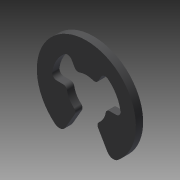
# Autodesk Inventor part: D-5406
Saved by Autodesk Inventor 2014 (Build 180170000, 170)
## iProperties
Created: 2014-01-19
Part Number: D-5406
Material: Generic
Catalog Web Link: www.cadenas.de
Description: Piston Rod Clevis for Original Line Cylinders - Retaining Ring-
Vendor: BIMBA
Document SubType Name: Standard Catalog Part
Designer: Michael
Manufacturer: BIMBA
Density: 1 g/cm^3
Appearance: RGB(84.00000259280115,84.00000259280115,84.00000259280115)
Category: PARTsolutions
Company: BIMBA
Title: D-5406
Author: Cadenas PARTsolutions
PSOL_IDENT_0: {$CADENAS_DATA\23d-libs\bimba\bimba\bimba_imperial\bimba_full_line\original_line_cylinders\accessori
PSOL_IDENT_1: es\piston_rod_clevis_rr.prj},210 {VTYP=3D},{NB=D-5406},{LINA=D-5406},{NN=Piston Rod Clevis for Origi
PSOL_IDENT_2: nal Line Cylinders - Retaining Ring},{DATE=06.12.2012 07:53:57},{GEOMDATE=06.12.2012 07:18:40},{VERS
PSOL_IDENT_3: ION=},{LINEID=20},{LINESUBID=-1},{WBVAR=}  {NB=D-5406},{LINA=D-5406},{KT=DUMMY},{PN=D-5406},{D=0.375
PSOL_IDENT_4: 00000},{D1=0.14850000},{D2=0.26175},{L=0.02750000},{COLOR=0.75,0.75,0.75,0.00}
CNS_NN: Piston Rod Clevis for Original Line Cylinders - Retaining Ring
CNS_NB: D-5406
CNS_NBSYN: $PN.
CNS_LINA: D-5406
CNS_PN: D-5406
CNS_D: 0.37500000
CNS_D1: 0.14850000
CNS_D2: 0.262
CNS_L: 0.02750000
CNS_COLOR: 0.75,0.75,0.75,0.00
SUPPLIER: BIMBA
ARTICLENO: D-5406
BOMINFO: D-5406
CREATOR: CADENAS GmbH
Autodesk Inventor part; units mm, degrees
ref_plane "YZ Plane" through (0, 0, 0) normal (1, 0, 0) x (0, 1, 0)
ref_plane "XZ Plane" through (0, 0, 0) normal (0, 1, 0) x (-1, 0, 0)
ref_plane "XY Plane" through (0, 0, 0) normal (0, 0, 1) x (1, 0, 0)
sketch "Sketch_1" plane through (0, 0, 0) normal (0, 0, 1) x (1, 0, 0)
  arc A0 (3.0189, -3.6834) -> (-3.0189, -3.6834) centre (0, 0) ccw
  arc A1 (-3.0189, -3.6834) -> (-2.0217, -3.5017) centre (-2.5975, -3.1692) ccw
  line L0 (-2.0217, -3.5017) -> (-1.1157, -1.9325)
  arc A2 (-1.1157, -1.9325) -> (-1.202, -1.4533) centre (-1.4424, -1.7439) ccw
  arc A3 (-1.8596, -0.3143) -> (-1.202, -1.4533) centre (0, 0) ccw
  arc A4 (-1.8596, -0.3143) -> (-2.2315, 0) centre (-2.2315, -0.3772) ccw
  line L1 (-2.2315, 0) -> (-2.8467, 0)
  arc A5 (-3.2846, 0.5114) -> (-2.8467, 0) centre (-2.8467, 0.4432) ccw
  arc A6 (-2.0852, 2.5889) -> (-3.2846, 0.5114) centre (0, 0) ccw
  arc A7 (-1.4233, 2.4653) -> (-2.0852, 2.5889) centre (-1.8072, 2.2437) ccw
  line L2 (-1.4233, 2.4653) -> (-1.1157, 1.9325)
  arc A8 (-1.1157, 1.9325) -> (-0.6576, 1.7676) centre (-0.7891, 2.1211) ccw
  arc A9 (0.6576, 1.7676) -> (-0.6576, 1.7676) centre (0, 0) ccw
  arc A10 (0.6576, 1.7676) -> (1.1157, 1.9325) centre (0.7891, 2.1211) ccw
  line L3 (1.1157, 1.9325) -> (1.4233, 2.4653)
  arc A11 (2.0852, 2.5889) -> (1.4233, 2.4653) centre (1.8072, 2.2437) ccw
  arc A12 (3.2846, 0.5114) -> (2.0852, 2.5889) centre (0, 0) ccw
  arc A13 (2.8467, 0) -> (3.2846, 0.5114) centre (2.8467, 0.4432) ccw
  line L4 (2.8467, 0) -> (2.2315, 0)
  arc A14 (2.2315, 0) -> (1.8596, -0.3143) centre (2.2315, -0.3772) ccw
  arc A15 (1.202, -1.4533) -> (1.8596, -0.3143) centre (0, 0) ccw
  arc A16 (1.202, -1.4533) -> (1.1157, -1.9325) centre (1.4424, -1.7439) ccw
  line L5 (1.1157, -1.9325) -> (2.0217, -3.5017)
  arc A17 (2.0217, -3.5017) -> (3.0189, -3.6834) centre (2.5975, -3.1692) ccw
  constraints: 36 point on circle, 18 centre point, 12 end point
extrude "Extrusion1" add sketch "Sketch_1" along normal mid plane 0.6985
ref_plane "RR_XY" through (0, 0, 0) normal (0, 0, 1) x (1, 0, 0)
ref_plane "RR_YZ" through (0, 0, 0) normal (1, 0, 0) x (0, 1, 0)
ref_plane "RR_ZX" through (0, 0, 0) normal (0, 1, 0) x (0, 0, 1)
body "Solid1"
